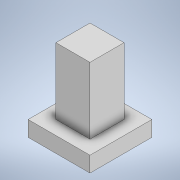
# Autodesk Inventor part: Button Prong
Saved by Autodesk Inventor 2021 (Build 250183000, 183)
## iProperties
Created: 2020-06-04
Part Number: Button Prong
Material: Generic
Document SubType Name: Modeling
Designer: ameli
Density: 1 g/cm^3
Appearance: Default
Author: ameli
Autodesk Inventor part; units mm, degrees
ref_plane "YZ Plane" through (0, 0, 0) normal (1, 0, 0) x (0, 1, 0)
ref_plane "XZ Plane" through (0, 0, 0) normal (0, 1, 0) x (-1, 0, 0)
ref_plane "XY Plane" through (0, 0, 0) normal (0, 0, 1) x (1, 0, 0)
sketch "Sketch1" plane through (0, 0, 0) normal (0, 1, 0) x (-1, 0, 0)
  line L0 (0, 0) -> (5.5, 0)
  line L1 (5.5, 0) -> (5.5, -5.5)
  line L2 (5.5, -5.5) -> (0, -5.5)
  line L3 (0, -5.5) -> (0, 0)
  dimension "d0" = 5.5
  dimension "d1" = 5.5
  constraints: 8 end point, 2 parallel, 1 horizontal, 1 perpendicular
  measures "d0" distance of L0.end L1.end
  measures "d1" distance of L1.end L2.end
extrude "Extrusion1" add sketch "Sketch1" along normal blind 10.75
sketch "Sketch2" plane through (0, 0, 0) normal (0, -1, 0) x (1, 0, 0)
  line L0 (-7.75, 2.25) -> (2.25, 2.25)
  line L1 (2.25, 2.25) -> (2.25, -7.75)
  line L2 (2.25, -7.75) -> (-7.75, -7.75)
  line L3 (-7.75, -7.75) -> (-7.75, 2.25)
  line L4 (-5.5, 0) -> (0, 0) projected
  line L5 (0, 0) -> (0, -5.5) projected
  dimension "d4" = 10
  dimension "d5" = 10
  dimension "d6" = 2.25
  dimension "d7" = 2.25
  constraints: 8 end point, 2 parallel, 1 horizontal, 1 perpendicular
  measures "d4" distance of L0.start L0.end
  measures "d5" distance of L0.end L1.end
  measures "d6" distance between parallel lines of L4 L0
  measures "d7" distance between parallel lines of L5 L1
extrude "Extrusion2" add sketch "Sketch2" along normal blind 2.5
body "Solid1"
